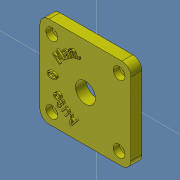
# Autodesk Inventor part: Schalter_Platte_Auto-Manuell
Saved by Autodesk Inventor 2019 (Build 230136000, 136)
## iProperties
Created: 2020-08-07
Part Number: Schalter_Platte_Auto-Manuell
Material: Generisch
Document SubType Name: Modeling
Designer: Stefan
Mass: 13.8091 g
Surface Area: 66.2174 cm^2
Volume: 13.8091 cm^3
Density: 1 g/cm^3
Appearance: Glatt - Gelb
Author: Stefan
Autodesk Inventor part; units mm, degrees
ref_plane "YZ Plane" through (0, 0, 0) normal (1, 0, 0) x (0, 1, 0)
ref_plane "XZ Plane" through (0, 0, 0) normal (0, 1, 0) x (-1, 0, 0)
ref_plane "XY Plane" through (0, 0, 0) normal (0, 0, 1) x (1, 0, 0)
sketch "Skizze1" plane through (0, 0, 0) normal (0, 0, 1) x (-1, 0, 0)
  line L0 (-20, 25) -> (20, 25)
  line L1 (25, 20) -> (25, -20)
  line L2 (20, -25) -> (-20, -25)
  line L3 (-25, -20) -> (-25, 20)
  line L4 (-25, 25) -> (25, -25) construction
  line L5 (25, 25) -> (-25, -25) construction
  arc A0 (25, 20) -> (20, 25) centre (20, 20) ccw
  arc A1 (20, -25) -> (25, -20) centre (20, -20) ccw
  arc A2 (-25, -20) -> (-20, -25) centre (-20, -20) ccw
  arc A3 (-20, 25) -> (-25, 20) centre (-20, 20) ccw
  circle A4 centre (0, 0) radius 5.5
  circle A5 centre (0, 0) radius 15 construction
  circle A6 centre (0, 0) radius 7.5
  line L6 (3.4517, 14.7516) -> (6.8343, 18.8013)
  line L7 (6.8343, 18.8013) -> (7.5971, 18.5047)
  line L8 (7.5971, 18.5047) -> (7.3567, 13.2338)
  line L9 (7.3567, 13.2338) -> (6.7034, 13.4877)
  line L10 (6.7034, 13.4877) -> (6.7868, 14.955)
  line L11 (6.7868, 14.955) -> (5.0081, 15.6465)
  line L12 (5.0081, 15.6465) -> (4.0786, 14.508)
  line L13 (4.0786, 14.508) -> (3.4517, 14.7516)
  line L14 (6.8224, 15.5498) -> (6.954, 18.0244)
  line L15 (6.954, 18.0244) -> (5.3835, 16.1091)
  line L16 (5.3835, 16.1091) -> (6.8224, 15.5498)
  line L17 (10.0895, 11.195) -> (9.5813, 11.5708)
  line L18 (9.5813, 11.5708) -> (9.8269, 11.9031)
  spline S0 degree 2 poles (9.8269, 11.9031) (9.4406, 11.8713) (8.8637, 11.9702) (8.6031, 12.1629) knots 0 0 0 1 2 2 2
  spline S1 degree 2 poles (8.6031, 12.1629) (8.4076, 12.3074) (8.1553, 12.6954) (8.1318, 12.9295) knots 0 0 0 1 2 2 2
  spline S2 degree 2 poles (8.1318, 12.9295) (8.105, 13.1659) (8.2772, 13.6987) (8.5036, 14.005) knots 0 0 0 1 2 2 2
  line L19 (8.5036, 14.005) -> (9.9511, 15.9632)
  line L20 (9.9511, 15.9632) -> (10.4594, 15.5875)
  line L21 (10.4594, 15.5875) -> (9.1877, 13.8671)
  spline S3 degree 2 poles (9.1877, 13.8671) (9.0095, 13.626) (8.8117, 13.2835) (8.7869, 13.1204) knots 0 0 0 1 2 2 2
  spline S4 degree 2 poles (8.7869, 13.1204) (8.7621, 12.9573) (8.8944, 12.6933) (9.0931, 12.5463) knots 0 0 0 1 2 2 2
  spline S5 degree 2 poles (9.0931, 12.5463) (9.2788, 12.409) (9.8557, 12.3101) (10.1449, 12.3332) knots 0 0 0 1 2 2 2
  line L22 (10.1449, 12.3332) -> (11.8116, 14.5879)
  line L23 (11.8116, 14.5879) -> (12.3199, 14.2122)
  line L24 (12.3199, 14.2122) -> (10.0895, 11.195)
  spline S6 degree 2 poles (11.4122, 9.632) (11.0688, 10.0152) (11.1197, 10.8388) (11.5935, 11.2633) knots 0 0 0 1 2 2 2
  line L25 (11.5935, 11.2633) -> (13.1416, 12.6504)
  line L26 (13.1416, 12.6504) -> (12.8577, 12.9672)
  line L27 (12.8577, 12.9672) -> (13.247, 13.316)
  line L28 (13.247, 13.316) -> (13.5309, 12.9992)
  line L29 (13.5309, 12.9992) -> (14.3336, 13.7184)
  line L30 (14.3336, 13.7184) -> (14.7554, 13.2476)
  line L31 (14.7554, 13.2476) -> (13.9527, 12.5284)
  line L32 (13.9527, 12.5284) -> (14.7287, 11.6623)
  line L33 (14.7287, 11.6623) -> (14.3394, 11.3135)
  line L34 (14.3394, 11.3135) -> (13.5634, 12.1796)
  line L35 (13.5634, 12.1796) -> (12.2326, 10.9872)
  spline S7 degree 2 poles (12.2326, 10.9872) (12.0213, 10.798) (11.8025, 10.5747) (11.7489, 10.4341) knots 0 0 0 1 2 2 2
  spline S8 degree 2 poles (11.7489, 10.4341) (11.6992, 10.3135) (11.782, 10.045) (11.928, 9.882) knots 0 0 0 1 2 2 2
  spline S9 degree 2 poles (11.928, 9.882) (12.0308, 9.7673) (12.2922, 9.6152) (12.3565, 9.5859) knots 0 0 0 1 2 2 2
  line L36 (12.3565, 9.5859) -> (12.3809, 9.5587)
  line L37 (12.3809, 9.5587) -> (11.9584, 9.1802)
  spline S10 degree 2 poles (11.9584, 9.1802) (11.8032, 9.2805) (11.5176, 9.5143) (11.4122, 9.632) knots 0 0 0 1 2 2 2
  spline S11 degree 2 poles (15.4059, 7.0898) (14.5879, 6.6103) (13.2355, 6.8742) (12.8503, 7.5314) knots 0 0 0 1 2 2 2
  spline S12 degree 2 poles (12.8503, 7.5314) (12.4548, 8.206) (12.9212, 9.5174) (13.7111, 9.9806) knots 0 0 0 1 2 2 2
  spline S13 degree 2 poles (13.7111, 9.9806) (14.5221, 10.456) (15.8876, 10.1857) (16.2688, 9.5356) knots 0 0 0 1 2 2 2
  spline S14 degree 2 poles (16.2688, 9.5356) (16.6541, 8.8784) (16.2203, 7.5673) (15.4059, 7.0898) knots 0 0 0 1 2 2 2
  spline S15 degree 2 poles (15.0759, 7.6526) (15.7051, 8.0215) (16.0484, 8.838) (15.8004, 9.2609) knots 0 0 0 1 2 2 2
  spline S16 degree 2 poles (15.8004, 9.2609) (15.5524, 9.6839) (14.6702, 9.7867) (14.0411, 9.4178) knots 0 0 0 1 2 2 2
  spline S17 degree 2 poles (14.0411, 9.4178) (13.4294, 9.0592) (13.0707, 8.2289) (13.3186, 7.806) knots 0 0 0 1 2 2 2
  spline S18 degree 2 poles (13.3186, 7.806) (13.5646, 7.3865) (14.4538, 7.2878) (15.0759, 7.6526) knots 0 0 0 1 2 2 2
  spline S19 degree 2 poles (17.5, -1.6005) (16.1548, -1.6005) (14.8947, -0.8185) (14.8947, -0.0041) knots 0 0 0 1 2 2 2
  spline S20 degree 2 poles (14.8947, -0.0041) (14.8947, 0.8225) (16.1791, 1.5964) (17.4959, 1.5964) knots 0 0 0 1 2 2 2
  spline S21 degree 2 poles (17.4959, 1.5964) (18.8493, 1.5964) (20.1013, 0.8144) (20.1013, -0.0041) knots 0 0 0 1 2 2 2
  spline S22 degree 2 poles (20.1013, -0.0041) (20.1013, -0.8266) (18.8047, -1.6005) (17.5, -1.6005) knots 0 0 0 1 2 2 2
  spline S23 degree 2 poles (15.9765, -0.7415) (16.2237, -0.8387) (16.9854, -0.9198) (17.5, -0.9198) knots 0 0 0 1 2 2 2
  spline S24 degree 2 poles (17.5, -0.9198) (18.0146, -0.9198) (18.7723, -0.8387) (19.0276, -0.7374) knots 0 0 0 1 2 2 2
  spline S25 degree 2 poles (19.0276, -0.7374) (19.2828, -0.6361) (19.5462, -0.2836) (19.5462, -0.0041) knots 0 0 0 1 2 2 2
  spline S26 degree 2 poles (19.5462, -0.0041) (19.5462, 0.2755) (19.2828, 0.6361) (19.0194, 0.7415) knots 0 0 0 1 2 2 2
  spline S27 degree 2 poles (19.0194, 0.7415) (18.7642, 0.8428) (17.9862, 0.9157) (17.4959, 0.9157) knots 0 0 0 1 2 2 2
  spline S28 degree 2 poles (17.4959, 0.9157) (16.9692, 0.9157) (16.2642, 0.8509) (15.9887, 0.7455) knots 0 0 0 1 2 2 2
  spline S29 degree 2 poles (15.9887, 0.7455) (15.7293, 0.6483) (15.4498, 0.2877) (15.4498, -0.0041) knots 0 0 0 1 2 2 2
  spline S30 degree 2 poles (15.4498, -0.0041) (15.4498, -0.2796) (15.7131, -0.6402) (15.9765, -0.7415) knots 0 0 0 1 2 2 2
  line L38 (10.711, -10.7177) -> (11.1098, -10.1862)
  line L39 (11.1098, -10.1862) -> (14.5548, -12.7714)
  line L40 (14.5548, -12.7714) -> (12.9948, -9.9695)
  line L41 (12.9948, -9.9695) -> (13.238, -9.6455)
  line L42 (13.238, -9.6455) -> (16.357, -10.37)
  line L43 (16.357, -10.37) -> (12.912, -7.7847)
  line L44 (12.912, -7.7847) -> (13.2841, -7.2889)
  line L45 (13.2841, -7.2889) -> (17.2832, -10.29)
  line L46 (17.2832, -10.29) -> (16.7385, -11.0159)
  line L47 (16.7385, -11.0159) -> (13.763, -10.3433)
  line L48 (13.763, -10.3433) -> (15.2647, -12.9799)
  line L49 (15.2647, -12.9799) -> (14.7102, -13.7188)
  line L50 (14.7102, -13.7188) -> (10.711, -10.7177)
  spline S31 degree 2 poles (8.5012, -12.8589) (8.5298, -12.7677) (8.6192, -12.451) (8.6813, -12.3301) knots 0 0 0 1 2 2 2
  spline S32 degree 2 poles (8.6813, -12.3301) (8.7626, -12.16) (8.9592, -11.9004) (9.188, -11.7328) knots 0 0 0 1 2 2 2
  spline S33 degree 2 poles (9.188, -11.7328) (9.3743, -11.5963) (9.8139, -11.4901) (10.0348, -11.5242) knots 0 0 0 1 2 2 2
  spline S34 degree 2 poles (10.0348, -11.5242) (10.2467, -11.5598) (10.662, -11.818) (10.8105, -12.0207) knots 0 0 0 1 2 2 2
  spline S35 degree 2 poles (10.8105, -12.0207) (11.0404, -12.3344) (11.1014, -12.9729) (10.9072, -13.3111) knots 0 0 0 1 2 2 2
  spline S36 degree 2 poles (10.9072, -13.3111) (10.7385, -13.6156) (10.1103, -14.2116) (9.725, -14.529) knots 0 0 0 1 2 2 2
  line L51 (9.725, -14.529) -> (9.7969, -14.6271)
  spline S37 degree 2 poles (9.7969, -14.6271) (9.9262, -14.8036) (10.1945, -14.9435) (10.3381, -14.9338) knots 0 0 0 1 2 2 2
  spline S38 degree 2 poles (10.3381, -14.9338) (10.4816, -14.924) (10.7915, -14.7573) (10.9418, -14.6471) knots 0 0 0 1 2 2 2
  spline S39 degree 2 poles (10.9418, -14.6471) (11.1183, -14.5178) (11.5188, -14.0635) (11.6832, -13.7874) knots 0 0 0 1 2 2 2
  line L52 (11.6832, -13.7874) -> (11.7126, -13.7658)
  line L53 (11.7126, -13.7658) -> (12.0934, -14.2855)
  spline S40 degree 2 poles (12.0934, -14.2855) (11.9816, -14.4277) (11.5272, -14.9113) (11.269, -15.1005) knots 0 0 0 1 2 2 2
  spline S41 degree 2 poles (11.269, -15.1005) (10.9553, -15.3304) (10.4553, -15.5461) (10.1919, -15.5432) knots 0 0 0 1 2 2 2
  spline S42 degree 2 poles (10.1919, -15.5432) (9.9342, -15.5411) (9.481, -15.2654) (9.2727, -14.9811) knots 0 0 0 1 2 2 2
  line L54 (9.2727, -14.9811) -> (7.7566, -12.9123)
  line L55 (7.7566, -12.9123) -> (8.2665, -12.5387)
  line L56 (8.2665, -12.5387) -> (8.5012, -12.8589)
  line L57 (8.8126, -13.2838) -> (9.4281, -14.1238)
  spline S43 degree 2 poles (9.4281, -14.1238) (9.5991, -13.9733) (10.1107, -13.513) (10.2456, -13.3338) knots 0 0 0 1 2 2 2
  spline S44 degree 2 poles (10.2456, -13.3338) (10.4028, -13.1232) (10.4783, -12.671) (10.3106, -12.4422) knots 0 0 0 1 2 2 2
  spline S45 degree 2 poles (10.3106, -12.4422) (10.119, -12.1808) (9.6309, -12.1316) (9.3498, -12.3375) knots 0 0 0 1 2 2 2
  spline S46 degree 2 poles (9.3498, -12.3375) (9.1112, -12.5124) (8.8699, -13.0057) (8.8126, -13.2838) knots 0 0 0 1 2 2 2
  line L58 (4.2632, -14.4581) -> (4.8489, -14.2204)
  line L59 (4.8489, -14.2204) -> (5.6535, -16.2027)
  spline S47 degree 2 poles (5.6535, -16.2027) (5.751, -16.443) (5.9637, -16.8377) (6.0815, -16.9342) knots 0 0 0 1 2 2 2
  spline S48 degree 2 poles (6.0815, -16.9342) (6.2062, -17.0366) (6.5133, -17.0606) (6.7311, -16.9723) knots 0 0 0 1 2 2 2
  spline S49 degree 2 poles (6.7311, -16.9723) (6.9488, -16.8839) (7.3161, -16.4637) (7.4615, -16.1861) knots 0 0 0 1 2 2 2
  line L60 (7.4615, -16.1861) -> (6.407, -13.588)
  line L61 (6.407, -13.588) -> (6.9927, -13.3503)
  line L62 (6.9927, -13.3503) -> (8.4037, -16.8269)
  line L63 (8.4037, -16.8269) -> (7.818, -17.0646)
  line L64 (7.818, -17.0646) -> (7.6611, -16.6779)
  spline S50 degree 2 poles (7.6611, -16.6779) (7.4943, -17.0211) (7.088, -17.4746) (6.8027, -17.5904) knots 0 0 0 1 2 2 2
  spline S51 degree 2 poles (6.8027, -17.5904) (6.2921, -17.7976) (5.4396, -17.3565) (5.179, -16.7145) knots 0 0 0 1 2 2 2
  line L65 (5.179, -16.7145) -> (4.2632, -14.4581)
  line L66 (2.4306, -14.8071) -> (3.2185, -14.6562)
  line L67 (3.2185, -14.6562) -> (3.3983, -15.5954)
  line L68 (3.3983, -15.5954) -> (2.6104, -15.7463)
  line L69 (2.6104, -15.7463) -> (2.4306, -14.8071)
  point P0 (18.5, 18.5)
  point P1 (18.5, -18.5)
  point P2 (-18.5, -18.5)
  point P3 (-18.5, 18.5)
  dimension "d0" = 50
  dimension "d1" = 50
  dimension "d2" = 5
  dimension "d5" = 37
  dimension "d13" = 11
  dimension "d14" = 30
  dimension "d17" = 15
  constraints: 12 end point, 12 point on line, 8 point on circle, 8 tangent, 7 centre point, 3 coincident, 3 equal radius, 2 horizontal alignment, 2 midpoint, 2 parallel, 1 horizontal, 1 perpendicular, 1 vertical alignment, 3 other
  measures "d0" distance of L5.start L4.end
  measures "d1" distance of L4.start L5.start
  measures "d2" radius of A0
  measures "d5" distance of point (18.5, -18.5) point (18.5, 18.5)
  measures "d13" diameter of A4
  measures "d14" diameter of A5
  measures "d17" diameter of A6
extrude "Extrusion1" add sketch "Skizze1" against normal blind 6 contours L0 A0 L1 A1 L2 A2 L3 A3 | A6 | L6 L7 L8 L9 L10 L11 L12 L13 | L16 L15 L14 | L17 L18 S0 S1 S2 L19 L20 L21 S3 S4 S5 L22 L23 L24 | S6 L25 L26 L27 L28 L29 L30 L31 L32 L33 L34 L35 S7 S8 S9 L36 L37 S10 | S11 S12 S13 S14 | S18 S17 S16 S15 | S19 S20 S21 S22 | S30 S29 S28 S27 S26 S25 S24 S23 | L38 L39 L40 L41 L42 L43 L44 L45 L46 L47 L48 L49 L50 | S31 S32 S33 S34 S35 S36 L51 S37 S38 S39 L52 L53 S40 S41 S42 L54 L55 L56 | S46 S45 S44 S43 L57 | L58 L59 S47 S48 S49 L60 L61 L62 L63 L64 S50 S51 L65 | L66 L67 L68 L69
emboss "Prägen1" sketch "Skizze1" operation add depth 1 direction (0, 0, -1) contours L6 L7 L8 L9 L10 L11 L12 L13 | L17 L18 S0 S1 S2 L19 L20 L21 S3 S4 S5 L22 L23 L24 | S6 L25 L26 L27 L28 L29 L30 L31 L32 L33 L34 L35 S7 S8 S9 L36 L37 S10 | S11 S12 S13 S14 | S19 S20 S21 S22 | L38 L39 L40 L41 L42 L43 L44 L45 L46 L47 L48 L49 L50 | S31 S32 S33 S34 S35 S36 L51 S37 S38 S39 L52 L53 S40 S41 S42 L54 L55 L56 | L58 L59 S47 S48 S49 L60 L61 L62 L63 L64 S50 S51 L65 | L66 L67 L68 L69
hole "Bohrung1" at (-18.5, -18.5, 0) at (-18.5, 18.5, 0) at (18.5, 18.5, 0) at (18.5, -18.5, 0) direction (0, 0, -1) diameter 3.4 end through all counterbore diameter 6.5 counterbore depth 3.4 clearance for "Inbusschraube DIN EN ISO 4762" size "M3" standard "DIN"
equation "\"d1\" = d0"
